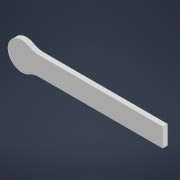
# Autodesk Inventor part: Рычаг_2
Saved by Autodesk Inventor 2021.2 (Build 252289000, 289)
## iProperties
Created: 2021-05-30
Part Number: Рычаг_2
Material: Типовые
Document SubType Name: Modeling
Designer: Admin
Density: 1 g/cm^3
Appearance: По умолчанию
Author: Admin
Autodesk Inventor part; units mm, degrees
ref_plane "YZ Plane" through (0, 0, 0) normal (1, 0, 0) x (0, 1, 0)
ref_plane "XZ Plane" through (0, 0, 0) normal (0, 1, 0) x (-1, 0, 0)
ref_plane "XY Plane" through (0, 0, 0) normal (0, 0, 1) x (1, 0, 0)
sketch "Эскиз1" plane through (0, 0, 0) normal (0, 0, 1) x (1, 0, 0)
  arc A0 (7.7262, 12.8571) -> (7.7262, -12.8571) centre (0, 0) ccw
  line L0 (18.0278, 10) -> (150, 10)
  line L1 (150, 10) -> (150, -10)
  line L2 (150, -10) -> (18.0278, -10)
  arc A1 (7.7262, 12.8571) -> (18.0278, 10) centre (18.0278, 30) ccw
  arc A2 (18.0278, -10) -> (7.7262, -12.8571) centre (18.0278, -30) ccw
  point P0 (11.1803, 10)
  point P1 (11.1803, -10)
  dimension "d0" = 30
  dimension "d1" = 150
  dimension "d13" = 20
  dimension "d14" = 10
  dimension "d15" = 20
  constraints: 8 point on circle, 6 end point, 4 tangent, 3 centre point, 2 horizontal, 2 point on line, 1 coincident, 1 equal radius, 1 vertical
  measures "d0" diameter of A0
  measures "d1" distance from line of L1 point (0, 0)
  measures "d13" distance between parallel lines of L2 L0
  measures "d14" distance from line of point (0, 0) L2
  measures "d15" radius of A1
extrude "Выдавливание1" add sketch "Эскиз1" along normal blind 5
sketch "Эскиз2" plane through (0, 0, 5) normal (0, 0, 1) x (1, 0, 0)
  arc A0 (7.7262, 12.8571) -> (7.7262, -12.8571) centre (0, 0) ccw projected
  circle A1 centre (0, 0) radius 5
  dimension "d16" = 10
  constraints: 2 coincident, 1 centre point
  measures "d16" diameter of A1
extrude "Выдавливание2" add sketch "Эскиз2" against normal blind 10
equation "\"d14\" = 0.5 * d13"
